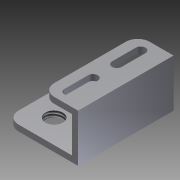
# Autodesk Inventor part: turn encoder mount
Saved by Autodesk Inventor 2012 (Build 160160000, 160)
## iProperties
Created: 2012-07-13
Part Number: turn encoder mount
Material: Default
Document SubType Name: Modeling
Designer: Bryce
Density: 1 g/cm^3
Author: Bryce
Autodesk Inventor part; units mm, degrees
ref_plane "YZ Plane" through (0, 0, 0) normal (1, 0, 0) x (0, 1, 0)
ref_plane "XZ Plane" through (0, 0, 0) normal (0, 1, 0) x (-1, 0, 0)
ref_plane "XY Plane" through (0, 0, 0) normal (0, 0, 1) x (1, 0, 0)
sketch "Sketch1" plane through (0, 0, 0) normal (0, 0, 1) x (1, 0, 0)
  line L0 (-19.05, 25.4) -> (0, 25.4)
  line L1 (0, 25.4) -> (0, 0)
  line L2 (-19.05, 25.4) -> (-19.05, 22.225)
  line L3 (-19.05, 22.225) -> (-3.175, 22.225)
  line L4 (-3.175, 22.225) -> (-3.175, 3.175)
  line L5 (-3.175, 3.175) -> (-38.1, 3.175)
  line L6 (-38.1, 3.175) -> (-38.1, 0)
  line L7 (-38.1, 0) -> (0, 0)
  dimension "d2" = 3.175
  dimension "d3" = 3.175
  dimension "d4" = 3.175
  dimension "d16" = 19.05
  dimension "d17" = 38.1
  dimension "d18" = 34.925
  dimension "d19" = 15.875
  dimension "d20" = 25.4
  constraints: 16 end point, 3 parallel, 2 perpendicular, 1 horizontal
  measures "d2" distance of L0.start L2.end
  measures "d3" distance of L5.end L6.end
  measures "d4" distance between parallel lines of L1 L4
  measures "d16" distance of L0.start L0.end
  measures "d17" distance of L6.end L1.end
  measures "d18" distance of L4.end L5.end
  measures "d19" distance of L2.end L3.end
  measures "d20" distance of L0.end L1.end
extrude "Extrusion1" add sketch "Sketch1" against normal blind 50.8
sketch "Sketch2" plane through (-38.1, 3.175, 0) normal (0, 1, 0) x (1, 0, 0)
  line L0 (34.925, 0) -> (0, 0) projected
  line L1 (34.925, 0) -> (34.925, 50.8) projected
  circle A0 centre (12.7, 12.7) radius 4.6482
  point P0 (38.1, 0)
  dimension "d9" = 9.2964
  dimension "d10" = 22.225
  dimension "d11" = 12.7
  constraints: 1 centre point
  measures "d9" diameter of A0
  measures "d10" distance from line of L1 A0.centre
  measures "d11" distance from line of L0 A0.centre
extrude "Extrusion2" cut sketch "Sketch2" against normal blind 50.8
thread "Thread1" size "3/8-16 UNC" class "2B" standard "ANSI Unified Screw Threads" full length
sketch "Sketch3" plane through (-19.05, 25.4, 0) normal (0, 1, 0) x (1, 0, 0)
  line L0 (19.05, 50.8) -> (0, 50.8) projected
  line L1 (0, 0) -> (0, 50.8) projected
  line L2 (19.05, 0) -> (19.05, 50.8) projected
  line L3 (5.3975, 19.05) -> (10.4775, 19.05)
  line L4 (10.4775, 19.05) -> (10.4775, 6.35)
  line L5 (10.4775, 6.35) -> (5.3975, 6.35)
  line L6 (5.3975, 6.35) -> (5.3975, 19.05)
  arc A0 (10.4775, 19.05) -> (5.3975, 19.05) centre (7.9375, 19.05) ccw
  arc A1 (5.3975, 6.35) -> (10.4775, 6.35) centre (7.9375, 6.35) ccw
  line L7 (5.3975, 44.45) -> (10.4775, 44.45)
  line L8 (10.4775, 44.45) -> (10.4775, 31.75)
  line L9 (10.4775, 31.75) -> (5.3975, 31.75)
  line L10 (5.3975, 31.75) -> (5.3975, 44.45)
  arc A2 (10.4775, 44.45) -> (5.3975, 44.45) centre (7.9375, 44.45) ccw
  arc A3 (5.3975, 31.75) -> (10.4775, 31.75) centre (7.9375, 31.75) ccw
  dimension "d21" = 12.7
  dimension "d22" = 5.08
  dimension "d23" = 31.75
  dimension "d24" = 11.1125
  dimension "d27" = 25.4
  constraints: 16 end point, 8 point on circle, 4 centre point, 4 tangent, 2 parallel, 1 horizontal, 1 perpendicular, 1 vertical, 12 other
  measures "d21" distance of L3.end L4.end
  measures "d22" distance of L4.end L5.end
  measures "d23" distance between parallel lines of L0 L3
  measures "d24" distance from line of L2 A1.centre
  measures "d27" distance of L3.start L7.start
extrude "Extrusion3" cut sketch "Sketch3" against normal blind 12.7
fillet "Fillet1" radius 6.35 4 edges at (-19.05, 23.8125, 0) (-38.1, 1.5875, 0) (-19.05, 23.8125, -50.8) (-38.1, 1.5875, -50.8)
body "Solid1"
